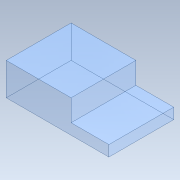
# Autodesk Inventor part: Blokje
Saved by Autodesk Inventor 2020.3 (Build 243373000, 373)
## iProperties
Created: 2020-10-24
Part Number: Blokje
Material: Generic
Document SubType Name: Modeling
Designer: Britt
Density: 1 g/cm^3
Appearance: Blue - Glazing
Author: Britt
Autodesk Inventor part; units mm, degrees
ref_plane "YZ Plane" through (0, 0, 0) normal (1, 0, 0) x (0, 1, 0)
ref_plane "XZ Plane" through (0, 0, 0) normal (0, 1, 0) x (-1, 0, 0)
ref_plane "XY Plane" through (0, 0, 0) normal (0, 0, 1) x (1, 0, 0)
sketch "Sketch1" plane through (0, 0, 0) normal (0, 1, 0) x (-1, 0, 0)
  line L0 (0, 0) -> (-95, 0)
  line L1 (-95, 0) -> (-95, -60)
  line L2 (-95, -60) -> (0, -60)
  line L3 (0, -60) -> (0, 0)
  dimension "d0" = 95
  dimension "d1" = 60
  constraints: 8 end point, 2 parallel, 1 horizontal, 1 perpendicular
  measures "d0" distance of L2.end L1.end
  measures "d1" distance of L1.end L0.end
extrude "Extrusion1" add sketch "Sketch1" along normal blind 30
sketch "Sketch2" plane through (0, 30, 0) normal (0, 1, 0) x (1, 0, 0)
  line L0 (0, 0) -> (95, 0) projected
  line L1 (0, 0) -> (60, 0)
  line L2 (60, 0) -> (95, 0)
  line L3 (95, 0) -> (95, 60) projected
  line L4 (95, 0) -> (95, 60)
  line L5 (95, 60) -> (60, 60)
  line L6 (95, 60) -> (0, 60) projected
  line L7 (60, 0) -> (60, 60)
  dimension "d4" = 60
  constraints: 10 end point, 2 perpendicular, 2 point on line, 1 collinear
  measures "d4" distance of L0.start L1.end
extrude "Extrusion2" cut sketch "Sketch2" against normal blind 20
body "Solid1"
